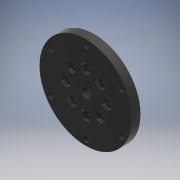
# Autodesk Inventor part: sea_connector
Saved by Autodesk Inventor 2018 (Build 220112000, 112)
## iProperties
Created: 2019-06-05
Part Number: sea_connector
Material: Generic
Document SubType Name: Modeling
Designer: Jasper
Density: 1 g/cm^3
Appearance: Default
Author: Jasper
Autodesk Inventor part; units mm, degrees
ref_plane "YZ Plane" through (0, 0, 0) normal (1, 0, 0) x (0, 1, 0)
ref_plane "XZ Plane" through (0, 0, 0) normal (0, 1, 0) x (-1, 0, 0)
ref_plane "XY Plane" through (0, 0, 0) normal (0, 0, 1) x (1, 0, 0)
sketch "Sketch1" plane through (0, 0, 0) normal (0, 1, 0) x (-1, 0, 0)
  circle A0 centre (0, 0) radius 25
  dimension "d0" = 50
  constraints: 1 centre point, 1 coincident
  measures "d0" diameter of A0
extrude "Extrusion1" add sketch "Sketch1" along normal blind 4.5
sketch "Sketch2" plane through (0, 4.5, 0) normal (0, 1, 0) x (1, 0, 0)
  line L0 (0, 0) -> (0, -22) construction
  circle A0 centre (0, -22) radius 1.6
  circle A1 centre (19.0526, -11) radius 1.6
  circle A2 centre (19.0526, 11) radius 1.6
  circle A3 centre (0, 22) radius 1.6
  circle A4 centre (-19.0526, 11) radius 1.6
  circle A5 centre (-19.0526, -11) radius 1.6
  dimension "d3" = 22
  dimension "d4" = 3.2
  dimension "d7" = 360
  constraints: 6 centre point, 2 end point, 1 coincident, 1 vertical, 13 other
  measures "d3" distance of L0.start L0.end
  measures "d4" diameter of A0
extrude "Extrusion2" cut sketch "Sketch2" against normal up to surface (4.5 mm away)
sketch "Sketch3" plane through (0, 4.5, 0) normal (0, 1, 0) x (1, 0, 0)
  line L0 (0, 0) -> (0, -11)
  line L1 (0, 0) -> (11, 0) construction
  circle A0 centre (0, -11) radius 1.35
  circle A1 centre (7.7782, -7.7782) radius 1.35
  circle A2 centre (11, 0) radius 1.35
  circle A3 centre (7.7782, 7.7782) radius 1.35
  circle A4 centre (0, 11) radius 1.35
  circle A5 centre (-7.7782, 7.7782) radius 1.35
  circle A6 centre (-11, 0) radius 1.35
  circle A7 centre (-7.7782, -7.7782) radius 1.35
  dimension "d11" = 11
  dimension "d12" = 90
  dimension "d13" = 2.7
  dimension "d16" = 360
  constraints: 8 centre point, 4 end point, 1 coincident, 1 horizontal, 1 perpendicular, 1 vertical, 17 other
  measures "d11" distance of L0.start L0.end
  measures "d12" angle of L0 L1
  measures "d13" diameter of A0
extrude "Extrusion3" cut sketch "Sketch3" against normal up to surface (4.5 mm away)
sketch "Sketch4" plane through (0, 0, 0) normal (0, -1, 0) x (1, 0, 0)
  circle A0 centre (-11, 0) radius 1.35 construction
  circle A1 centre (-7.7782, 7.7782) radius 1.35 construction
  circle A2 centre (-7.7782, -7.7782) radius 1.35 construction
  circle A3 centre (7.7782, -7.7782) radius 1.35 construction
  circle A4 centre (7.7782, 7.7782) radius 1.35 construction
  circle A5 centre (0, 11) radius 1.35 construction
  circle A6 centre (11, 0) radius 1.35 construction
  circle A7 centre (0, -11) radius 1.35 construction
  circle A8 centre (-19.0526, -11) radius 1.6 construction
  circle A9 centre (-19.0526, 11) radius 1.6 construction
  circle A10 centre (0, -22) radius 1.6 construction
  circle A11 centre (19.0526, 11) radius 1.6 construction
  circle A12 centre (0, 22) radius 1.6 construction
  circle A13 centre (19.0526, -11) radius 1.6 construction
  circle A14 centre (0, 0) radius 25 construction
  line L0 (0, 0) -> (0, -8.5) construction
  line L1 (1.4434, -8.5) -> (2.8868, -11)
  line L2 (2.8868, -11) -> (1.4434, -13.5)
  line L3 (1.4434, -13.5) -> (-1.4434, -13.5)
  line L4 (-1.4434, -13.5) -> (-2.8868, -11)
  line L5 (-2.8868, -11) -> (-1.4434, -8.5)
  line L6 (-1.4434, -8.5) -> (1.4434, -8.5)
  line L7 (5.7369, -9.8194) -> (4.9898, -7.031)
  line L8 (8.5253, -10.5666) -> (5.7369, -9.8194)
  line L9 (10.5666, -8.5253) -> (8.5253, -10.5666)
  line L10 (9.8194, -5.7369) -> (10.5666, -8.5253)
  line L11 (7.031, -4.9898) -> (9.8194, -5.7369)
  line L12 (4.9898, -7.031) -> (7.031, -4.9898)
  line L13 (11, -2.8868) -> (8.5, -1.4434)
  line L14 (13.5, -1.4434) -> (11, -2.8868)
  line L15 (13.5, 1.4434) -> (13.5, -1.4434)
  line L16 (11, 2.8868) -> (13.5, 1.4434)
  line L17 (8.5, 1.4434) -> (11, 2.8868)
  line L18 (8.5, -1.4434) -> (8.5, 1.4434)
  line L19 (9.8194, 5.7369) -> (7.031, 4.9898)
  line L20 (10.5666, 8.5253) -> (9.8194, 5.7369)
  line L21 (8.5253, 10.5666) -> (10.5666, 8.5253)
  line L22 (5.7369, 9.8194) -> (8.5253, 10.5666)
  line L23 (4.9898, 7.031) -> (5.7369, 9.8194)
  line L24 (7.031, 4.9898) -> (4.9898, 7.031)
  line L25 (2.8868, 11) -> (1.4434, 8.5)
  line L26 (1.4434, 13.5) -> (2.8868, 11)
  line L27 (-1.4434, 13.5) -> (1.4434, 13.5)
  line L28 (-2.8868, 11) -> (-1.4434, 13.5)
  line L29 (-1.4434, 8.5) -> (-2.8868, 11)
  line L30 (1.4434, 8.5) -> (-1.4434, 8.5)
  line L31 (-5.7369, 9.8194) -> (-4.9898, 7.031)
  line L32 (-8.5253, 10.5666) -> (-5.7369, 9.8194)
  line L33 (-10.5666, 8.5253) -> (-8.5253, 10.5666)
  line L34 (-9.8194, 5.7369) -> (-10.5666, 8.5253)
  line L35 (-7.031, 4.9898) -> (-9.8194, 5.7369)
  line L36 (-4.9898, 7.031) -> (-7.031, 4.9898)
  line L37 (-11, 2.8868) -> (-8.5, 1.4434)
  line L38 (-13.5, 1.4434) -> (-11, 2.8868)
  line L39 (-13.5, -1.4434) -> (-13.5, 1.4434)
  line L40 (-11, -2.8868) -> (-13.5, -1.4434)
  line L41 (-8.5, -1.4434) -> (-11, -2.8868)
  line L42 (-8.5, 1.4434) -> (-8.5, -1.4434)
  line L43 (-9.8194, -5.7369) -> (-7.031, -4.9898)
  line L44 (-10.5666, -8.5253) -> (-9.8194, -5.7369)
  line L45 (-8.5253, -10.5666) -> (-10.5666, -8.5253)
  line L46 (-5.7369, -9.8194) -> (-8.5253, -10.5666)
  line L47 (-4.9898, -7.031) -> (-5.7369, -9.8194)
  line L48 (-7.031, -4.9898) -> (-4.9898, -7.031)
  point P0 (6.0104, -6.0104)
  point P1 (8.5, 0)
  point P2 (6.0104, 6.0104)
  point P3 (0, 8.5)
  point P4 (-6.0104, 6.0104)
  point P5 (-8.5, 0)
  point P6 (-6.0104, -6.0104)
  dimension "d20" = 8.5
  dimension "d23" = 360
  constraints: 98 end point, 1 coincident, 1 midpoint, 1 vertical, 118 other
  measures "d20" distance of L0.start L0.end
extrude "Extrusion4" cut sketch "Sketch4" against normal blind 2
sketch "Sketch5" plane through (0, 4.5, 0) normal (0, 1, 0) x (1, 0, 0)
  circle A0 centre (-11, 0) radius 1.35 construction
  circle A1 centre (-7.7782, -7.7782) radius 1.35 construction
  circle A2 centre (-7.7782, 7.7782) radius 1.35 construction
  circle A3 centre (7.7782, 7.7782) radius 1.35 construction
  circle A4 centre (7.7782, -7.7782) radius 1.35 construction
  circle A5 centre (0, -11) radius 1.35 construction
  circle A6 centre (11, 0) radius 1.35 construction
  circle A7 centre (0, 11) radius 1.35 construction
  circle A8 centre (-19.0526, 11) radius 1.6 construction
  circle A9 centre (-19.0526, -11) radius 1.6 construction
  circle A10 centre (0, 22) radius 1.6 construction
  circle A11 centre (19.0526, -11) radius 1.6 construction
  circle A12 centre (0, -22) radius 1.6 construction
  circle A13 centre (19.0526, 11) radius 1.6 construction
  circle A14 centre (0, 0) radius 25 construction
  circle A15 centre (0, -22) radius 2.35
  circle A16 centre (19.0526, -11) radius 2.35
  circle A17 centre (19.0526, 11) radius 2.35
  circle A18 centre (0, 22) radius 2.35
  circle A19 centre (-19.0526, 11) radius 2.35
  circle A20 centre (-19.0526, -11) radius 2.35
  dimension "d27" = 4.7
  dimension "d30" = 360
  constraints: 6 centre point, 1 coincident, 13 other
  measures "d27" diameter of A15
extrude "Extrusion5" cut sketch "Sketch5" against normal blind 2.6
sketch "Sketch6" plane through (0, 4.5, 0) normal (0, 1, 0) x (1, 0, 0)
  circle A0 centre (0, 0) radius 2.8
  dimension "d34" = 5.6
  constraints: 1 centre point, 1 coincident
  measures "d34" diameter of A0
extrude "Extrusion6" cut sketch "Sketch6" against normal up to surface (4.5 mm away)
sketch "Sketch7" plane through (0, 4.5, 0) normal (0, 1, 0) x (1, 0, 0)
  circle A0 centre (0, 0) radius 2.8 construction
  circle A1 centre (-19.0526, 11) radius 2.35 construction
  circle A2 centre (19.0526, 11) radius 2.35 construction
  circle A3 centre (0, -22) radius 2.35 construction
  circle A4 centre (19.0526, -11) radius 2.35 construction
  circle A5 centre (0, 22) radius 2.35 construction
  circle A6 centre (-19.0526, -11) radius 2.35 construction
  circle A7 centre (-11, 0) radius 1.35 construction
  circle A8 centre (-7.7782, -7.7782) radius 1.35 construction
  circle A9 centre (-7.7782, 7.7782) radius 1.35 construction
  circle A10 centre (7.7782, 7.7782) radius 1.35 construction
  circle A11 centre (7.7782, -7.7782) radius 1.35 construction
  circle A12 centre (0, -11) radius 1.35 construction
  circle A13 centre (11, 0) radius 1.35 construction
  circle A14 centre (0, 11) radius 1.35 construction
  circle A15 centre (0, 0) radius 25 construction
  line L0 (0, -22) -> (0, -18) construction
  line L1 (0, -18) -> (2.1213, -15.8787)
  line L2 (0, -18) -> (3, -18) construction
  line L3 (2.1213, -15.8787) -> (0.6213, -15.8787)
  line L4 (0.6213, -15.8787) -> (0.6213, -12.8787)
  line L5 (0.6213, -12.8787) -> (0.2071, -12.8787)
  line L6 (0, -18) -> (-2.1213, -15.8787)
  line L7 (-2.1213, -15.8787) -> (-0.6213, -15.8787)
  line L8 (-0.6213, -15.8787) -> (-0.6213, -12.8787)
  line L9 (-0.6213, -12.8787) -> (0.2071, -12.8787)
  dimension "d37" = 4
  dimension "d38" = 3
  dimension "d39" = 45
  dimension "d40" = 1.5
  dimension "d41" = 45
  dimension "d42" = 3
  constraints: 20 end point, 3 symmetric about line, 2 horizontal, 2 vertical, 1 equal length, 1 perpendicular
  measures "d37" distance of L0.start L0.end
  measures "d38" distance of L0.end L1.end
  measures "d39" angle of L2 L1
  measures "d40" distance of L1.end L3.end
  measures "d41" angle of L3 L1
  measures "d42" distance of L3.end L4.end
extrude "Extrusion7" cut sketch "Sketch7" against normal blind 0.4
body "Solid1"
